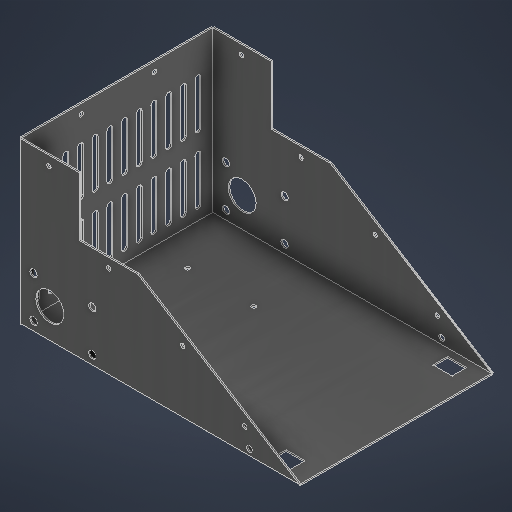
# Autodesk Inventor part: qveda_korpusi
Saved by Autodesk Inventor 2026.2 (Build 302298000, 298)
## iProperties
Created: 2026-03-05
Part Number: qveda_korpusi
Material: Generic
Document SubType Name: Sheet Metal
Designer: User
Density: 1 g/cm^3
Sheet Metal Rule: Default_mm
Appearance: Dark Gray
Flat Pattern Width: 29.9692 cm
Flat Pattern Length: 34.9383 cm
Flat Pattern Area: 1047.07 cm^2
Sheet Metal Width: 299.692 mm
Sheet Metal Length: 349.383 mm
Sheet Metal Area: 104707.325 mm^2
Author: User
Autodesk Inventor part; units mm, degrees
ref_plane "YZ Plane" through (0, 0, 0) normal (1, 0, 0) x (0, 1, 0)
ref_plane "XZ Plane" through (0, 0, 0) normal (0, 1, 0) x (-1, 0, 0)
ref_plane "XY Plane" through (0, 0, 0) normal (0, 0, 1) x (1, 0, 0)
sketch "Sketch1" plane through (0, 0, 0) normal (0, 1, 0) x (-1, 0, 0)
  line L0 (181.4219, 127.0802) -> (-8.5781, 127.0802)
  line L1 (-8.5781, 127.0802) -> (-8.5781, -2.9198)
  line L2 (-8.5781, -2.9198) -> (181.4219, -2.9198)
  line L3 (181.4219, -2.9198) -> (181.4219, 127.0802)
  point P0 (0, 0)
  dimension "d0" = 190
  dimension "d1" = 130
  measures "d0" distance of L2.end L1.end
  measures "d1" distance of L1.end L0.end
extrude "Plate1" add sketch "Sketch1" along normal blind 1
sketch "Sketch2" plane through (-181.4229, 1.001, 127.0802) normal (-1, 0, 0) x (0, -1, 0)
  line L0 (0, -130) -> (0, 0)
  line L1 (0, 0) -> (-108.999, 0)
  line L2 (-108.999, 0) -> (-108.999, -130)
  line L3 (-108.999, -130) -> (0, -130)
  constraints: 6 end point, 1 horizontal, 1 perpendicular, 1 vertical
edge flange "Flange1" height 110 angle 90 thickness 1 bend radius 0 thickness toward (-1, 0, 0) relief round relief width 1 relief depth 0.5 edges at (-181.4219, 1, 62.0802) wall of the first edge with corners at (-181.4229, 1.001, -2.9198) (-181.4229, 1.001, 127.0802) (-181.4229, 110, 127.0802) (-181.4229, 110, -2.9198)
bend "Bend1"
corner "Corner1"
sketch "Sketch3" plane through (8.5781, 1.001, 127.0812) normal (0, 0, 1) x (1, 0, 0)
  line L0 (-190, 0) -> (0, 0)
  line L1 (0, 0) -> (0, 108.999)
  line L2 (0, 108.999) -> (-190, 108.999)
  line L3 (-190, 108.999) -> (-190, 0)
  constraints: 6 end point, 1 horizontal, 1 perpendicular, 1 vertical
edge flange "Flange2" height 110 angle 90 thickness 1 bend radius 0 thickness toward (0, 0, 1) relief straight relief width 1 relief depth 0.5 edges at (-86.4224, 1, 127.0802) wall of the first edge with corners at (-181.4219, 1.001, 127.0812) (8.5781, 1.001, 127.0812) (8.5781, 110, 127.0812) (-181.4219, 110, 127.0812)
bend "Bend2"
corner "Corner2"
sketch "Sketch4" plane through (-181.4219, 1.001, -2.9208) normal (0, 0, -1) x (-1, 0, 0)
  line L0 (-190, 0) -> (0, 0)
  line L1 (0, 0) -> (0, 108.999)
  line L2 (0, 108.999) -> (-190, 108.999)
  line L3 (-190, 108.999) -> (-190, 0)
  constraints: 6 end point, 1 horizontal, 1 perpendicular, 1 vertical
edge flange "Flange3" height 110 angle 90 thickness 1 bend radius 0 thickness toward (0, 0, -1) relief straight relief width 1 relief depth 0.5 edges at (-86.4224, 1, -2.9198) wall of the first edge with corners at (8.5781, 1.001, -2.9208) (-181.4219, 1.001, -2.9208) (-181.4219, 110, -2.9208) (8.5781, 110, -2.9208)
bend "Bend3"
corner "Corner3"
sketch "Sketch5" plane through (-181.4219, 110, 128.0812) normal (0, 0, 1) x (1, 0, 0)
  line L0 (190, -108.999) -> (0, -108.999) projected
  line L1 (190, 0) -> (0, 0) projected
  line L2 (9.8667, 0) -> (190, 0)
  line L3 (190, -108.999) -> (190, 0) projected
  line L4 (190, -108.999) -> (190, 0)
  line L5 (0, 0) -> (190, 0) projected
  line L6 (0, 0) -> (50, 0)
  line L7 (50, 0) -> (50, 0)
  line L8 (50, 0) -> (0, 0)
  line L9 (0, 0) -> (0, 0)
  line L10 (50, 0) -> (190, 0)
  line L11 (190, 0) -> (190, 0)
  line L12 (190, 0) -> (50, 0)
  line L13 (50, 0) -> (50, 0)
  line L14 (0, 0) -> (40, 0)
  line L15 (40, 0) -> (40, -40)
  line L16 (40, -40) -> (0, -40)
  line L17 (0, -40) -> (0, 0)
  line L18 (40, -40) -> (190, -40)
  line L19 (190, -40) -> (190, 0)
  line L20 (190, 0) -> (40, 0)
  line L21 (40, 0) -> (40, -40)
  line L22 (40, -40) -> (80, -40)
  line L23 (80, -40) -> (80, 0)
  line L24 (80, 0) -> (40, 0)
  line L25 (40, 0) -> (40, -40)
  line L26 (80, -40) -> (190, -108.999)
  point P0 (181.4219, -110)
  point P1 (40, 0)
  point P2 (190, 0)
  point P3 (80, -40)
  point P4 (190, -40)
  dimension "d39" = 50
  dimension "d40" = 40
  dimension "d41" = 40
  dimension "d44" = 40
  dimension "d45" = 40
  constraints: 46 end point, 8 parallel, 5 horizontal, 5 perpendicular, 4 collinear, 2 point on line
  measures "d39" distance of L8.end L7.end
  measures "d40" distance of L15.end L16.end
  measures "d41" distance of L14.end L15.end
  measures "d44" distance of L24.end L23.end
  measures "d45" distance of L23.end L22.end
extrude "Cut1" cut sketch "Sketch5" against normal blind 1 contours L3 L18 L23 L1 | L23 L18 L15 L1 | L3 L26 L18
sketch "Sketch6" plane through (8.5781, 110, -3.9208) normal (0, 0, -1) x (-1, 0, 0)
  line L0 (0, 0) -> (0, -108.999) projected
  line L1 (0, 0) -> (190, 0) projected
  line L2 (0, -34.999) -> (0, -108.999)
  line L3 (0, -108.999) -> (190, -108.999) projected
  line L4 (190, 0) -> (150, 0)
  line L5 (150, 0) -> (150, -40)
  line L6 (150, -40) -> (190, -40)
  line L7 (190, -40) -> (190, 0)
  line L8 (150, -40) -> (0, -40)
  line L9 (0, -40) -> (0, 0)
  line L10 (0, 0) -> (150, 0)
  line L11 (150, 0) -> (150, -40)
  line L12 (150, -40) -> (110, -40)
  line L13 (110, -40) -> (110, 0)
  line L14 (110, 0) -> (150, 0)
  line L15 (150, 0) -> (150, -40)
  line L16 (0, -108.999) -> (110, -40)
  point P0 (8.5781, -110)
  point P1 (150, 0)
  point P2 (110, -40)
  point P3 (0, -40)
  dimension "d42" = 40
  dimension "d43" = 40
  dimension "d46" = 40
  dimension "d47" = 40
  constraints: 28 end point, 6 parallel, 3 horizontal, 3 perpendicular, 1 vertical
  measures "d42" distance of L6.end L5.end
  measures "d43" distance of L5.end L4.end
  measures "d46" distance of L13.end L14.end
  measures "d47" distance of L12.end L13.end
extrude "Cut2" cut sketch "Sketch6" against normal blind 1 contours L1 L13 L8 L0 | L1 L5 L8 L13 | L8 L16 L0
sketch "Sketch8" plane through (-182.4229, 110, -2.9198) normal (-1, 0, 0) x (0, 0, 1)
  line L0 (10, -99.999) -> (10, -69.999) construction
  line L1 (12, -99.999) -> (12, -69.999)
  line L2 (8, -69.999) -> (8, -99.999)
  arc A0 (8, -99.999) -> (12, -99.999) centre (10, -99.999) ccw
  arc A1 (12, -69.999) -> (8, -69.999) centre (10, -69.999) ccw
  line L3 (0, -108.999) -> (0, 0) projected
  line L4 (0, -108.999) -> (130, -108.999) projected
  line L5 (20, -99.999) -> (20, -69.999) construction
  line L6 (22, -99.999) -> (22, -69.999)
  line L7 (18, -69.999) -> (18, -99.999)
  arc A2 (18, -99.999) -> (22, -99.999) centre (20, -99.999) ccw
  arc A3 (22, -69.999) -> (18, -69.999) centre (20, -69.999) ccw
  line L8 (30, -99.999) -> (30, -69.999) construction
  line L9 (32, -99.999) -> (32, -69.999)
  line L10 (28, -69.999) -> (28, -99.999)
  arc A4 (28, -99.999) -> (32, -99.999) centre (30, -99.999) ccw
  arc A5 (32, -69.999) -> (28, -69.999) centre (30, -69.999) ccw
  line L11 (40, -99.999) -> (40, -69.999) construction
  line L12 (42, -99.999) -> (42, -69.999)
  line L13 (38, -69.999) -> (38, -99.999)
  arc A6 (38, -99.999) -> (42, -99.999) centre (40, -99.999) ccw
  arc A7 (42, -69.999) -> (38, -69.999) centre (40, -69.999) ccw
  line L14 (50, -99.999) -> (50, -69.999) construction
  line L15 (52, -99.999) -> (52, -69.999)
  line L16 (48, -69.999) -> (48, -99.999)
  arc A8 (48, -99.999) -> (52, -99.999) centre (50, -99.999) ccw
  arc A9 (52, -69.999) -> (48, -69.999) centre (50, -69.999) ccw
  line L17 (60, -99.999) -> (60, -69.999) construction
  line L18 (62, -99.999) -> (62, -69.999)
  line L19 (58, -69.999) -> (58, -99.999)
  arc A10 (58, -99.999) -> (62, -99.999) centre (60, -99.999) ccw
  arc A11 (62, -69.999) -> (58, -69.999) centre (60, -69.999) ccw
  line L20 (70, -99.999) -> (70, -69.999) construction
  line L21 (72, -99.999) -> (72, -69.999)
  line L22 (68, -69.999) -> (68, -99.999)
  arc A12 (68, -99.999) -> (72, -99.999) centre (70, -99.999) ccw
  arc A13 (72, -69.999) -> (68, -69.999) centre (70, -69.999) ccw
  line L23 (80, -99.999) -> (80, -69.999) construction
  line L24 (82, -99.999) -> (82, -69.999)
  line L25 (78, -69.999) -> (78, -99.999)
  arc A14 (78, -99.999) -> (82, -99.999) centre (80, -99.999) ccw
  arc A15 (82, -69.999) -> (78, -69.999) centre (80, -69.999) ccw
  line L26 (90, -99.999) -> (90, -69.999) construction
  line L27 (92, -99.999) -> (92, -69.999)
  line L28 (88, -69.999) -> (88, -99.999)
  arc A16 (88, -99.999) -> (92, -99.999) centre (90, -99.999) ccw
  arc A17 (92, -69.999) -> (88, -69.999) centre (90, -69.999) ccw
  line L29 (100, -99.999) -> (100, -69.999) construction
  line L30 (102, -99.999) -> (102, -69.999)
  line L31 (98, -69.999) -> (98, -99.999)
  arc A18 (98, -99.999) -> (102, -99.999) centre (100, -99.999) ccw
  arc A19 (102, -69.999) -> (98, -69.999) centre (100, -69.999) ccw
  line L32 (110, -99.999) -> (110, -69.999) construction
  line L33 (112, -99.999) -> (112, -69.999)
  line L34 (108, -69.999) -> (108, -99.999)
  arc A20 (108, -99.999) -> (112, -99.999) centre (110, -99.999) ccw
  arc A21 (112, -69.999) -> (108, -69.999) centre (110, -69.999) ccw
  line L35 (120, -99.999) -> (120, -69.999) construction
  line L36 (122, -99.999) -> (122, -69.999)
  line L37 (118, -69.999) -> (118, -99.999)
  arc A22 (118, -99.999) -> (122, -99.999) centre (120, -99.999) ccw
  arc A23 (122, -69.999) -> (118, -69.999) centre (120, -69.999) ccw
  line L38 (10, -54.999) -> (10, -24.999) construction
  line L39 (12, -54.999) -> (12, -24.999)
  line L40 (8, -24.999) -> (8, -54.999)
  arc A24 (8, -54.999) -> (12, -54.999) centre (10, -54.999) ccw
  arc A25 (12, -24.999) -> (8, -24.999) centre (10, -24.999) ccw
  line L41 (20, -54.999) -> (20, -24.999) construction
  line L42 (22, -54.999) -> (22, -24.999)
  line L43 (18, -24.999) -> (18, -54.999)
  arc A26 (18, -54.999) -> (22, -54.999) centre (20, -54.999) ccw
  arc A27 (22, -24.999) -> (18, -24.999) centre (20, -24.999) ccw
  line L44 (30, -54.999) -> (30, -24.999) construction
  line L45 (32, -54.999) -> (32, -24.999)
  line L46 (28, -24.999) -> (28, -54.999)
  arc A28 (28, -54.999) -> (32, -54.999) centre (30, -54.999) ccw
  arc A29 (32, -24.999) -> (28, -24.999) centre (30, -24.999) ccw
  line L47 (40, -54.999) -> (40, -24.999) construction
  line L48 (42, -54.999) -> (42, -24.999)
  line L49 (38, -24.999) -> (38, -54.999)
  arc A30 (38, -54.999) -> (42, -54.999) centre (40, -54.999) ccw
  arc A31 (42, -24.999) -> (38, -24.999) centre (40, -24.999) ccw
  line L50 (50, -54.999) -> (50, -24.999) construction
  line L51 (52, -54.999) -> (52, -24.999)
  line L52 (48, -24.999) -> (48, -54.999)
  arc A32 (48, -54.999) -> (52, -54.999) centre (50, -54.999) ccw
  arc A33 (52, -24.999) -> (48, -24.999) centre (50, -24.999) ccw
  line L53 (60, -54.999) -> (60, -24.999) construction
  line L54 (62, -54.999) -> (62, -24.999)
  line L55 (58, -24.999) -> (58, -54.999)
  arc A34 (58, -54.999) -> (62, -54.999) centre (60, -54.999) ccw
  arc A35 (62, -24.999) -> (58, -24.999) centre (60, -24.999) ccw
  line L56 (70, -54.999) -> (70, -24.999) construction
  line L57 (72, -54.999) -> (72, -24.999)
  line L58 (68, -24.999) -> (68, -54.999)
  arc A36 (68, -54.999) -> (72, -54.999) centre (70, -54.999) ccw
  arc A37 (72, -24.999) -> (68, -24.999) centre (70, -24.999) ccw
  line L59 (80, -54.999) -> (80, -24.999) construction
  line L60 (82, -54.999) -> (82, -24.999)
  line L61 (78, -24.999) -> (78, -54.999)
  arc A38 (78, -54.999) -> (82, -54.999) centre (80, -54.999) ccw
  arc A39 (82, -24.999) -> (78, -24.999) centre (80, -24.999) ccw
  line L62 (90, -54.999) -> (90, -24.999) construction
  line L63 (92, -54.999) -> (92, -24.999)
  line L64 (88, -24.999) -> (88, -54.999)
  arc A40 (88, -54.999) -> (92, -54.999) centre (90, -54.999) ccw
  arc A41 (92, -24.999) -> (88, -24.999) centre (90, -24.999) ccw
  line L65 (100, -54.999) -> (100, -24.999) construction
  line L66 (102, -54.999) -> (102, -24.999)
  line L67 (98, -24.999) -> (98, -54.999)
  arc A42 (98, -54.999) -> (102, -54.999) centre (100, -54.999) ccw
  arc A43 (102, -24.999) -> (98, -24.999) centre (100, -24.999) ccw
  line L68 (110, -54.999) -> (110, -24.999) construction
  line L69 (112, -54.999) -> (112, -24.999)
  line L70 (108, -24.999) -> (108, -54.999)
  arc A44 (108, -54.999) -> (112, -54.999) centre (110, -54.999) ccw
  arc A45 (112, -24.999) -> (108, -24.999) centre (110, -24.999) ccw
  line L71 (120, -54.999) -> (120, -24.999) construction
  line L72 (122, -54.999) -> (122, -24.999)
  line L73 (118, -24.999) -> (118, -54.999)
  arc A46 (118, -54.999) -> (122, -54.999) centre (120, -54.999) ccw
  arc A47 (122, -24.999) -> (118, -24.999) centre (120, -24.999) ccw
  circle A48 centre (39.5, -6.5) radius 1.5
  circle A49 centre (89.5, -6.5) radius 1.5
  line L74 (0, 0) -> (130, 0) projected
  line L75 (130, 0) -> (130, -108.999) projected
  point P0 (2.9198, -110)
  point P1 (10, -84.999)
  point P2 (10, -101.999)
  point P3 (20, -101.999)
  point P4 (20, -84.999)
  point P5 (30, -101.999)
  point P6 (30, -84.999)
  point P7 (40, -101.999)
  point P8 (40, -84.999)
  point P9 (50, -101.999)
  point P10 (50, -84.999)
  point P11 (60, -101.999)
  point P12 (60, -84.999)
  point P13 (70, -101.999)
  point P14 (70, -84.999)
  point P15 (80, -101.999)
  point P16 (80, -84.999)
  point P17 (90, -101.999)
  point P18 (90, -84.999)
  point P19 (100, -101.999)
  point P20 (100, -84.999)
  point P21 (110, -101.999)
  point P22 (110, -84.999)
  point P23 (120, -101.999)
  point P24 (120, -84.999)
  point P25 (10, -56.999)
  point P26 (10, -39.999)
  point P27 (20, -56.999)
  point P28 (20, -39.999)
  point P29 (30, -56.999)
  point P30 (30, -39.999)
  point P31 (40, -56.999)
  point P32 (40, -39.999)
  point P33 (50, -56.999)
  point P34 (50, -39.999)
  point P35 (60, -56.999)
  point P36 (60, -39.999)
  point P37 (70, -56.999)
  point P38 (70, -39.999)
  point P39 (80, -56.999)
  point P40 (80, -39.999)
  point P41 (90, -56.999)
  point P42 (90, -39.999)
  point P43 (100, -56.999)
  point P44 (100, -39.999)
  point P45 (110, -56.999)
  point P46 (110, -39.999)
  point P47 (120, -56.999)
  point P48 (120, -39.999)
  dimension "d48" = 4
  dimension "d49" = 10
  dimension "d50" = 7
  dimension "d53" = 10
  dimension "d56" = 45
  dimension "d95" = 30
  dimension "d96" = 3
  dimension "d97" = 3
  dimension "d98" = 6.5
  dimension "d99" = 6.5
  dimension "d100" = 40.5
  dimension "d101" = 50
  constraints: 192 end point, 97 point on circle, 50 centre point, 4 tangent, 2 vertical, 1 horizontal, 1 midpoint, 1 parallel, 299 other
  measures "d48" diameter of A1
  measures "d49" distance between parallel lines of L3 L0
  measures "d50" distance from line of L4 point (10, -101.999)
  measures "d53" distance of L1.start L6.start
  measures "d56" distance of L1.start L39.start
  measures "d95" distance of L2.start L2.end
  measures "d96" diameter of A48
  measures "d97" diameter of A49
  measures "d98" distance from line of L74 A49.centre
  measures "d99" distance from line of L74 A48.centre
  measures "d100" distance from line of L75 A49.centre
  measures "d101" distance of A49.centre A48.centre
extrude "Cut3" cut sketch "Sketch8" against normal blind 1 contours A0 L2 A1 L1 | A2 L7 A3 L6 | A4 L10 A5 L9 | A6 L13 A7 L12 | A8 L16 A9 L15 | A10 L19 A11 L18 | A12 L22 A13 L21 | A14 L25 A15 L24 | A16 L28 A17 L27 | A18 L31 A19 L30 | A20 L34 A21 L33 | A22 L37 A23 L36 | A24 L40 A25 L39 | A26 L43 A27 L42 | A28 L46 A29 L45 | A30 L49 A31 L48 | A32 L52 A33 L51 | A34 L55 A35 L54 | A36 L58 A37 L57 | A38 L61 A39 L60 | A40 L64 A41 L63 | A42 L67 A43 L66 | A44 L70 A45 L69 | A48 | A49
sketch "Sketch9" plane through (-181.4219, 1.001, 128.0812) normal (0, 0, 1) x (1, 0, 0)
  line L0 (0, 0) -> (190, 0) projected
  line L1 (0, 0) -> (58, 0)
  line L2 (58, 0) -> (58, 40)
  line L3 (58, 40) -> (0, 40)
  line L4 (0, 40) -> (0, 0)
  line L5 (0, 20) -> (58, 20)
  line L6 (29, 40) -> (29, 0)
  circle A0 centre (9, 34) radius 2.5
  circle A1 centre (9, 6) radius 2.5
  circle A2 centre (49, 34) radius 2.5
  circle A3 centre (49, 6) radius 2.5
  circle A4 centre (20.1, 20) radius 9.5
  point P0 (181.4219, -1.001)
  point P1 (29, 16.6774)
  point P2 (29, 23.3226)
  dimension "d61" = 58
  dimension "d62" = 40
  dimension "d63" = 5
  dimension "d64" = 40
  dimension "d65" = 28
  dimension "d66" = 19
  dimension "d67" = 20.1
  constraints: 12 end point, 5 centre point, 4 midpoint, 3 symmetric about line, 2 parallel, 1 horizontal, 1 perpendicular, 1 point on line, 3 other
  measures "d61" distance of L3.end L2.end
  measures "d62" distance of L2.end L1.end
  measures "d63" diameter of A0
  measures "d64" diameter of A0.centre L6
  measures "d65" diameter of A0.centre L5
  measures "d66" diameter of A4
  measures "d67" distance from line of L4 A4.centre
ref_plane "Work Plane1" through (-181.4219, 1.001, 62.0802) normal (0, 0, 1) x (1, 0, 0)
extrude "Cut4" cut sketch "Sketch9" against normal blind 1 contours A4 L5 L6 | L6 L5 A4 | A4 L6 L5 | L6 A4 L5 | A0 | A1 | A2 | A3
mirror "Mirror1" about plane through (-181.4219, 1.001, 62.0802) normal (0, 0, 1) of "Cut4"
sketch "Sketch10" plane through (0, 1, 0) normal (0, 1, 0) x (1, 0, 0)
  line L0 (-3.4219, -122.0812) -> (-16.4219, -122.0812)
  line L1 (-16.4219, -122.0812) -> (-16.4219, -112.0812)
  line L2 (-16.4219, -112.0812) -> (-3.4219, -112.0812)
  line L3 (-3.4219, -112.0812) -> (-3.4219, -122.0812)
  line L4 (-101.4219, -127.0812) -> (8.5781, -127.0812) projected
  line L5 (8.5781, 2.9198) -> (8.5781, -127.0802) projected
  line L6 (-181.4229, -127.0802) -> (-181.4229, 2.9198) projected
  line L7 (-181.4229, -62.0802) -> (8.5781, -62.0802)
  line L8 (-3.4219, -2.0792) -> (-16.4219, -2.0792)
  line L9 (-16.4219, -2.0792) -> (-16.4219, -12.0792)
  line L10 (-16.4219, -12.0792) -> (-3.4219, -12.0792)
  line L11 (-3.4219, -12.0792) -> (-3.4219, -2.0792)
  point P0 (0, 0)
  dimension "d70" = 13
  dimension "d71" = 10
  dimension "d72" = 5
  dimension "d73" = 12
  constraints: 18 end point, 4 symmetric about line, 2 midpoint, 2 parallel, 1 horizontal, 1 perpendicular
  measures "d70" distance of L1.end L2.end
  measures "d71" distance of L0.end L1.end
  measures "d72" distance between parallel lines of L4 L0
  measures "d73" distance between parallel lines of L5 L3
extrude "Cut5" cut sketch "Sketch10" against normal blind 1
sketch "Sketch11" plane through (-181.4219, 1.001, 128.0812) normal (0, 0, 1) x (1, 0, 0)
  circle A0 centre (156, 4) radius 2
  line L0 (0, 0) -> (190, 0) projected
  circle A1 centre (60.2, 62.499) radius 1.5
  circle A2 centre (110.6432, 42.1047) radius 1.5
  circle A3 centre (152.8724, 15.6159) radius 1.5
  line L1 (190, 0) -> (80, 68.999) projected
  line L2 (80, 68.999) -> (40, 68.999) projected
  line L3 (40, 68.999) -> (40, 108.999) projected
  line L4 (80, 68.999) -> (70.402, 53.6976)
  line L5 (190, 0) -> (192.7111, 4.3221)
  circle A4 centre (19.5, 102.499) radius 1.5
  line L6 (0, 108.999) -> (40, 108.999) projected
  point P0 (181.4219, -1.001)
  dimension "d76" = 4
  dimension "d77" = 4
  dimension "d78" = 34
  dimension "d81" = 3
  dimension "d82" = 3
  dimension "d83" = 3
  dimension "d84" = 6.5
  dimension "d85" = 6.5
  dimension "d86" = 6.5
  dimension "d88" = 20.2
  dimension "d89" = 79.5
  dimension "d90" = 80.5
  dimension "d91" = 90
  dimension "d92" = 3
  dimension "d93" = 6.5
  dimension "d94" = 20.5
  constraints: 5 centre point, 4 end point, 1 perpendicular
  measures "d76" diameter of A0
  measures "d77" distance from line of L0 A0.centre
  measures "d78" horizontal distance of L0.end A0.centre
  measures "d81" diameter of A1
  measures "d82" diameter of A2
  measures "d83" diameter of A3
  measures "d84" distance from line of L1 A3.centre
  measures "d85" distance from line of L1 A2.centre
  measures "d86" distance from line of L2 A1.centre
  measures "d88" distance from line of A1.centre L3
  measures "d89" diameter of A3.centre L5
  measures "d90" diameter of A2.centre L4
  measures "d91" angle of L4 L1
  measures "d92" diameter of A4
  measures "d93" distance from line of L6 A4.centre
  measures "d94" distance from line of L3 A4.centre
extrude "Cut6" cut sketch "Sketch11" against normal blind 1
mirror "Mirror2" about plane through (-181.4219, 1.001, 62.0802) normal (0, 0, 1) of "Cut6"
sketch "Sketch12" plane through (0, 1, 0) normal (0, 1, 0) x (1, 0, 0)
  circle A0 centre (-156.9229, -38.5792) radius 1.5
  line L0 (-181.4229, 2.9198) -> (-181.4229, -127.0802) projected
  line L1 (-141.4219, 2.9208) -> (-181.4219, 2.9208) projected
  circle A1 centre (-156.9229, -83.5792) radius 1.5
  circle A2 centre (-111.9229, -83.5792) radius 1.5
  circle A3 centre (-111.9229, -38.5792) radius 1.5
  line L2 (-101.4219, 2.9208) -> (-141.4219, 2.9208) projected
  point P0 (0, 0)
  dimension "d102" = 3
  dimension "d103" = 24.5
  dimension "d104" = 41.5
  dimension "d105" = 3
  dimension "d106" = 3
  dimension "d107" = 3
  dimension "d108" = 24.5
  dimension "d109" = 45
  dimension "d110" = 45
  dimension "d111" = 45
  dimension "d112" = 45
  dimension "d113" = 41.5
  constraints: 4 centre point
  measures "d102" diameter of A0
  measures "d103" distance from line of L0 A0.centre
  measures "d104" distance from line of L1 A0.centre
  measures "d105" diameter of A1
  measures "d106" diameter of A2
  measures "d107" diameter of A3
  measures "d108" distance from line of L0 A1.centre
  measures "d109" distance of A1.centre A0.centre
  measures "d110" distance of A1.centre A2.centre
  measures "d111" distance of A3.centre A0.centre
  measures "d112" distance of A2.centre A3.centre
  measures "d113" distance from line of L2 A3.centre
extrude "Cut7" cut sketch "Sketch12" against normal blind 1
sketch "Sketch13" plane through (-182.4229, 110, -2.9198) normal (-1, 0, 0) x (0, 0, 1)
  line L0 (117.25, -23) -> (122.75, -23)
  line L1 (122.75, -23) -> (122.75, -31.9)
  line L2 (121.25, -33.4) -> (118.75, -33.4)
  line L3 (117.25, -31.9) -> (117.25, -23)
  line L4 (118.75, -33.4) -> (117.25, -31.9)
  line L5 (122.75, -31.9) -> (121.25, -33.4)
  line L6 (0, 0) -> (130, 0) projected
  line L7 (130, 0) -> (130, -108.999) projected
  line L8 (120, -54.999) -> (120, -39.3178) construction
  line L9 (122, -54.999) -> (122, -39.3178)
  line L10 (118, -39.3178) -> (118, -54.999)
  arc A0 (118, -54.999) -> (122, -54.999) centre (120, -54.999) ccw
  arc A1 (122, -39.3178) -> (118, -39.3178) centre (120, -39.3178) ccw
  arc A2 (122, -69.999) -> (118, -69.999) centre (120, -69.999) ccw projected
  point P0 (2.9198, -110)
  point P1 (122.75, -33.4)
  point P2 (117.25, -33.4)
  point P3 (120, -47.1584)
  dimension "d116" = 5.5
  dimension "d117" = 10.4
  dimension "d118" = 1.5
  dimension "d119" = 1.5
  dimension "d120" = 1.5
  dimension "d121" = 1.5
  dimension "d122" = 23
  dimension "d123" = 7.25
  dimension "d124" = 4
  dimension "d125" = 8
  dimension "d126" = 15
  constraints: 20 end point, 4 point on circle, 4 point on line, 4 tangent, 3 parallel, 2 centre point, 1 horizontal, 1 midpoint, 1 perpendicular, 1 vertical
  measures "d116" distance of point (122.75, -33.4) point (117.25, -33.4)
  measures "d117" distance of L0.end point (122.75, -33.4)
  measures "d118" distance of L2.end point (117.25, -33.4)
  measures "d119" distance of L3.start point (117.25, -33.4)
  measures "d120" distance of L1.end point (122.75, -33.4)
  measures "d121" distance of L2.start point (122.75, -33.4)
  measures "d122" distance between parallel lines of L6 L0
  measures "d123" distance between parallel lines of L7 L1
  measures "d124" diameter of A1
  measures "d125" distance between parallel lines of L7 L9
  measures "d126" distance of A2.centre L8.start
extrude "Cut8" cut sketch "Sketch13" against normal blind 1
equation "\"d34\" = Thickness"
equation "\"d37\" = Thickness"
equation "\"d59\" = Thickness"
equation "\"d68\" = Thickness"
equation "\"d74\" = Thickness"
equation "\"d79\" = Thickness"
equation "\"d114\" = Thickness"
equation "\"d2\" = Thickness"
equation "\"d3\" = BendReliefWidth"
equation "\"d4\" = BendReliefDepth"
equation "\"d5\" = MinimumRemnant"
equation "\"d10\" = CornerReliefSize"
equation "\"d11\" = GapSize"
equation "\"d13\" = BendReliefWidth"
equation "\"d14\" = BendReliefDepth"
equation "\"d15\" = MinimumRemnant"
equation "\"d20\" = CornerReliefSize"
equation "\"d21\" = GapSize"
equation "\"d23\" = BendReliefWidth"
equation "\"d24\" = BendReliefDepth"
equation "\"d25\" = MinimumRemnant"
equation "\"d30\" = CornerReliefSize"
equation "\"d31\" = GapSize"
equation "\"d119\" = d118"
equation "\"d120\" = d118"
equation "\"d121\" = d120"
equation "\"BendReliefWidth\" = Thickness"
equation "\"BendReliefDepth\" = 0.5 * Thickness"
equation "\"CornerReliefSize\" = 4 * Thickness"
equation "\"MinimumRemnant\" = 2 * Thickness"
equation "\"GapSize\" = Thickness"
equation "\"Thickness\" = 1"
body "Solid1"
